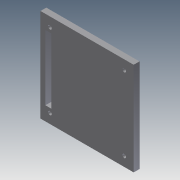
# Autodesk Inventor part: kinect rotate2 side
Saved by Autodesk Inventor 2011 (Build 150239000, 239)
## iProperties
Created: 2011-09-17
Part Number: kinect rotate2 side
Document SubType Name: Modeling
Designer: Matthew
Density: 1 g/cm^3
Author: Matthew
Autodesk Inventor part; units mm, degrees
ref_plane "YZ Plane" through (0, 0, 0) normal (1, 0, 0) x (0, 1, 0)
ref_plane "XZ Plane" through (0, 0, 0) normal (0, 1, 0) x (-1, 0, 0)
ref_plane "XY Plane" through (0, 0, 0) normal (0, 0, 1) x (1, 0, 0)
sketch "Sketch1" plane through (0, 0, 0) normal (0, 0, 1) x (1, 0, 0)
  line L0 (-25.4072, 25.3665) -> (76.1928, 25.3665)
  line L1 (76.1928, 25.3665) -> (76.1928, -76.2335)
  line L2 (76.1928, -76.2335) -> (-25.4072, -76.2335)
  line L3 (-25.4072, -76.2335) -> (-25.4072, 25.3665)
  point P0 (0, 0)
  dimension "d0" = 101.6
  dimension "d1" = 101.6
  constraints: 8 end point, 2 parallel, 1 horizontal, 1 perpendicular
  measures "d0" distance of L1.end L2.end
  measures "d1" distance of L0.end L1.end
extrude "Extrusion1" add sketch "Sketch1" along normal blind 0.7366
sketch "Sketch2" plane through (0, 0, 0.7366) normal (0, 0, 1) x (1, 0, 0)
  line L0 (-25.4072, 25.3665) -> (76.1928, -76.2335)
  line L1 (76.1928, 25.3665) -> (-25.4072, -76.2335)
  circle A0 centre (25.3928, -25.4335) radius 27.432
  point P0 (0, 0)
  dimension "d4" = 54.864
  constraints: 4 end point, 1 centre point, 1 midpoint, 1 perpendicular
  measures "d4" diameter of A0
extrude "Extrusion2" cut sketch "Sketch2" against normal blind 0.7366
sketch "Sketch3" plane through (0, 0, 0.7366) normal (0, 0, 1) x (1, 0, 0)
  line L0 (-25.4072, -76.2335) -> (-25.4072, 25.3665) projected
  line L1 (-25.4072, 25.3665) -> (-25.4072, -25.4335)
  line L2 (-25.4072, -25.4335) -> (-25.4072, 19.4102)
  line L3 (-25.4072, 25.3665) -> (76.1928, -76.2335)
  line L4 (76.1928, 25.3665) -> (-25.4072, -76.2335)
  circle A0 centre (-19.4509, 19.4102) radius 1.9812
  point P0 (0, 0)
  dimension "d7" = 44.8437
  dimension "d8" = 3.9624
  constraints: 8 end point, 2 point on line, 1 centre point, 1 midpoint, 1 perpendicular
  measures "d7" distance of L1.end L2.end
  measures "d8" diameter of A0
extrude "Extrusion3" cut sketch "Sketch3" against normal blind 0.7366 contours A0 L3 | L3 A0
sketch "Sketch4" plane through (0, 0, 0.7366) normal (0, 0, 1) x (1, 0, 0)
  line L0 (-25.4072, -76.2335) -> (76.1928, 25.3665)
  line L1 (-25.4072, 25.3665) -> (76.1928, -76.2335)
  circle A0 centre (70.2365, 19.4102) radius 1.9819
  circle A1 centre (70.2365, -70.2772) radius 1.983
  circle A2 centre (-19.4509, -70.2772) radius 1.9812
  point P0 (0, 0)
  constraints: 4 end point, 3 centre point, 3 point on line, 1 perpendicular
extrude "Extrusion4" cut sketch "Sketch4" against normal blind 0.7366
sketch "Sketch5" plane through (0, 0, 0.7366) normal (0, 0, 1) x (1, 0, 0)
  circle A0 centre (25.3928, -25.4335) radius 27.432 projected
  circle A1 centre (25.3928, -25.4335) radius 29.972
  circle A2 centre (25.3928, -25.4335) radius 32.512
  point P0 (0, 0)
  dimension "d13" = 59.944
  dimension "d14" = 65.024
  constraints: 2 centre point, 2 coincident
  measures "d13" diameter of A1
  measures "d14" diameter of A2
extrude "Extrusion5" add sketch "Sketch5" along normal blind 6.6548 contours A2
fillet "Fillet1" radius 3.175 4 edges at (-25.4072, 25.3665, 0.3683) (76.1928, 25.3665, 0.3683) (76.1928, -76.2335, 0.3683) (-25.4072, -76.2335, 0.3683)
sketch "Sketch6" plane through (25.3928, -25.4335, 0.7366) normal (0, 0, 1) x (1, 0, 0)
  circle A0 centre (0, 0) radius 29.972 projected
  circle A1 centre (0, 0) radius 27.432 projected
  point P0 (-25.3928, 25.4335)
extrude "Extrusion6" add sketch "Sketch6" along normal blind 9.1948
sketch "Sketch7" plane through (25.3928, -25.4335, 7.3914) normal (0, 0, 1) x (1, 0, 0)
  circle A0 centre (0, 0) radius 29.972 projected
  circle A1 centre (0, 0) radius 32.512 projected
  point P0 (-25.3928, 25.4335)
extrude "Extrusion7" cut sketch "Sketch7" against normal blind 6.6548
sketch "Sketch8" plane through (25.3928, -25.4335, 9.9314) normal (0, 0, 1) x (1, 0, 0)
  circle A0 centre (0, 0) radius 27.432 projected
  circle A1 centre (0, 0) radius 29.972 projected
  point P0 (-25.3928, 25.4335)
extrude "Extrusion8" cut sketch "Sketch8" against normal blind 2.54
sketch "Sketch9" plane through (0, 0, 0.7366) normal (0, 0, 1) x (1, 0, 0)
  circle A0 centre (-19.4509, 19.4102) radius 1.9812 projected
  circle A1 centre (70.2365, -70.2772) radius 1.983 projected
  circle A2 centre (-19.4509, -70.2772) radius 1.9812 projected
  circle A3 centre (70.2365, 19.4102) radius 1.9819 projected
  point P0 (0, 0)
extrude "Extrusion9" add sketch "Sketch9" against normal blind 0.7366
sketch "Sketch10" plane through (0, 0, 0.7366) normal (0, 0, 1) x (1, 0, 0)
  line L0 (-25.4072, 25.3665) -> (76.1928, 25.3665)
  line L1 (76.1928, 25.3665) -> (76.1928, -76.2335)
  line L2 (76.1928, -76.2335) -> (-25.4072, -76.2335)
  line L3 (-25.4072, -76.2335) -> (-25.4072, 25.3665)
  line L4 (-25.4072, 25.3665) -> (76.1928, -76.2335)
  line L5 (-25.4072, -76.2335) -> (76.1928, 25.3665)
  line L6 (-25.4072, 25.3665) -> (-25.4072, -25.4335)
  line L7 (-25.4072, -25.4335) -> (-25.4072, 15.0541)
  circle A0 centre (-15.0948, 15.0541) radius 1.9812
  circle A1 centre (65.8804, 15.0541) radius 1.9818
  circle A2 centre (65.8804, -65.9211) radius 1.9832
  circle A3 centre (-15.0948, -65.9211) radius 1.9812
  point P0 (0, 0)
  dimension "d26" = 40.4876
  dimension "d27" = 3.9624
  constraints: 16 end point, 5 point on line, 4 centre point, 2 parallel, 2 perpendicular, 1 horizontal, 1 midpoint
  measures "d26" distance of L6.end L7.end
  measures "d27" diameter of A0
extrude "Extrusion10" cut sketch "Sketch10" against normal blind 0.7366 contours A0 L4 | L4 A0 | A1 L5 | L5 A1 | A2 L4 | L4 A2 | A3 L5 | L5 A3
sketch "Sketch11" plane through (0, 0, 0.7366) normal (0, 0, 1) x (1, 0, 0)
  circle A0 centre (-15.0948, 15.0541) radius 1.9812 projected
  circle A1 centre (-15.0948, -65.9211) radius 1.9812 projected
  circle A2 centre (65.8804, 15.0541) radius 1.9818 projected
  circle A3 centre (65.8804, -65.9211) radius 1.9832 projected
  line L0 (-25.4072, 25.3665) -> (76.1928, 25.3665)
  line L1 (76.1928, 25.3665) -> (76.1928, -76.2335)
  line L2 (76.1928, -76.2335) -> (-25.4072, -76.2335)
  line L3 (-25.4072, -76.2335) -> (-25.4072, 25.3665)
  point P0 (0, 0)
  constraints: 8 end point, 2 parallel, 1 horizontal, 1 perpendicular
extrude "Extrusion11" add sketch "Sketch11" along normal blind 12.7
sketch "Sketch12" plane through (0, 0, 13.4366) normal (0, 0, 1) x (1, 0, 0)
  circle A0 centre (65.8804, -65.9211) radius 1.9832 projected
  circle A1 centre (65.8804, 15.0541) radius 1.9818 projected
  circle A2 centre (-15.0948, 15.0541) radius 1.9812 projected
  circle A3 centre (-15.0948, -65.9211) radius 1.9812 projected
  line L0 (76.1928, 25.3665) -> (76.1928, -76.2335) projected
  line L1 (-25.4072, 25.3665) -> (76.1928, 25.3665) projected
  line L2 (-25.4072, -76.2335) -> (-25.4072, 25.3665) projected
  line L3 (76.1928, -76.2335) -> (-25.4072, -76.2335) projected
  point P0 (0, 0)
extrude "Extrusion12" add sketch "Sketch12" against normal blind 19.05
sketch "Sketch13" plane through (0, 0, 13.4366) normal (0, 0, 1) x (1, 0, 0)
  circle A0 centre (65.8804, -65.9211) radius 1.9832 projected
  circle A1 centre (65.8804, 15.0541) radius 1.9818 projected
  circle A2 centre (-15.0948, 15.0541) radius 1.9812 projected
  circle A3 centre (-15.0948, -65.9211) radius 1.9812 projected
  line L0 (76.1928, 25.3665) -> (76.1928, -76.2335) projected
  line L1 (-25.4072, 25.3665) -> (76.1928, 25.3665) projected
  line L2 (-25.4072, -76.2335) -> (-25.4072, 25.3665) projected
  line L3 (76.1928, -76.2335) -> (-25.4072, -76.2335) projected
  point P0 (0, 0)
extrude "Extrusion13" cut sketch "Sketch13" against normal blind 12.7
sketch "Sketch14" plane through (-25.4072, 25.3665, -5.6134) normal (0, 1, 0) x (1, 0, 0)
  line L0 (0, -6.35) -> (101.6, -6.35) projected
  line L1 (101.6, -6.35) -> (101.6, 0) projected
  line L2 (101.6, 0) -> (0, 0) projected
  line L3 (0, 0) -> (0, -6.35) projected
  point P0 (25.4072, -5.6134)
sketch "Sketch15" plane through (-25.4072, -76.2335, -5.6134) normal (-1, 0, 0) x (0, 0, 1)
  line L0 (6.35, 0) -> (6.35, 101.6) projected
  line L1 (0, 101.6) -> (6.35, 101.6) projected
  line L2 (0, 101.6) -> (0, 0) projected
  line L3 (6.35, 0) -> (0, 0) projected
  point P0 (5.6134, 76.2335)
sketch "Sketch16" plane through (-25.4072, -76.2335, -5.6134) normal (0, -1, 0) x (1, 0, 0)
  line L0 (101.6, 6.35) -> (0, 6.35) projected
  line L1 (0, 6.35) -> (0, 0) projected
  line L2 (0, 0) -> (101.6, 0) projected
  line L3 (101.6, 6.35) -> (101.6, 0) projected
  point P0 (25.4072, 5.6134)
sketch "Sketch17" plane through (76.1928, -76.2335, -5.6134) normal (1, 0, 0) x (0, 0, -1)
  line L0 (-6.35, 101.6) -> (-6.35, 0) projected
  line L1 (-6.35, 0) -> (0, 0) projected
  line L2 (0, 0) -> (0, 101.6) projected
  line L3 (-6.35, 101.6) -> (0, 101.6) projected
  point P0 (-5.6134, 76.2335)
extrude "Extrusion14" add sketch "Sketch14" along normal blind 53.975
extrude "Extrusion15" add sketch "Sketch17" along normal blind 47.625
extrude "Extrusion16" add sketch "Sketch16" along normal blind 47.625
extrude "Extrusion17" add sketch "Sketch15" along normal blind 53.975
sketch "Sketch18" plane through (-25.4072, 25.3665, 0.7366) normal (0, 1, 0) x (1, 0, 0)
  line L0 (-53.975, 6.35) -> (-53.975, 0) projected
  line L1 (0, 0) -> (-53.975, 0) projected
  line L2 (0, 6.35) -> (0, 0) projected
  line L3 (0, 6.35) -> (-53.975, 6.35) projected
  point P0 (25.4072, 0.7366)
extrude "Extrusion18" add sketch "Sketch18" along normal blind 53.975
sketch "Sketch19" plane through (76.1928, 25.3665, 0.7366) normal (0, 1, 0) x (1, 0, 0)
  line L0 (47.625, 0) -> (47.625, 6.35) projected
  line L1 (0, 6.35) -> (47.625, 6.35) projected
  line L2 (0, 0) -> (0, 6.35) projected
  line L3 (0, 0) -> (47.625, 0) projected
  point P0 (-76.1928, 0.7366)
extrude "Extrusion19" add sketch "Sketch19" along normal blind 53.975
sketch "Sketch20" plane through (-25.4072, -123.8585, -5.6134) normal (-1, 0, 0) x (0, 0, 1)
  line L0 (6.35, 47.625) -> (0, 47.625) projected
  line L1 (0, 47.625) -> (0, 0) projected
  line L2 (0, 0) -> (6.35, 0) projected
  line L3 (6.35, 0) -> (6.35, 47.625) projected
  point P0 (5.6134, 123.8585)
extrude "Extrusion20" add sketch "Sketch20" along normal blind 53.975
sketch "Sketch21" plane through (123.8178, -76.2335, -5.6134) normal (0, -1, 0) x (1, 0, 0)
  line L0 (-47.625, 6.35) -> (-47.625, 0) projected
  line L1 (-47.625, 0) -> (0, 0) projected
  line L2 (0, 0) -> (0, 6.35) projected
  line L3 (0, 6.35) -> (-47.625, 6.35) projected
  point P0 (-123.8178, 5.6134)
extrude "Extrusion21" add sketch "Sketch21" along normal blind 47.625
sketch "Sketch22" plane through (-25.4072, 79.3415, -5.6134) normal (0, 1, 0) x (1, 0, 0)
  line L0 (149.225, -6.35) -> (-53.975, -6.35) projected
  line L1 (149.225, 0) -> (149.225, -6.35) projected
  line L2 (-53.975, 0) -> (149.225, 0) projected
  line L3 (-53.975, -6.35) -> (-53.975, 0) projected
  point P0 (25.4072, -5.6134)
extrude "Extrusion22" cut sketch "Sketch22" against normal blind 53.975
sketch "Sketch23" plane through (-79.3822, -76.2335, -5.6134) normal (-1, 0, 0) x (0, 0, 1)
  line L0 (6.35, 101.6) -> (0, 101.6) projected
  line L1 (0, -47.625) -> (0, 101.6) projected
  line L2 (6.35, -47.625) -> (0, -47.625) projected
  line L3 (6.35, 101.6) -> (6.35, -47.625) projected
  point P0 (5.6134, 76.2335)
extrude "Extrusion23" cut sketch "Sketch23" against normal blind 53.975
sketch "Sketch24" plane through (-25.4072, -123.8585, -5.6134) normal (0, -1, 0) x (1, 0, 0)
  line L0 (0, 6.35) -> (0, 0) projected
  line L1 (149.225, 0) -> (0, 0) projected
  line L2 (149.225, 6.35) -> (149.225, 0) projected
  line L3 (0, 6.35) -> (149.225, 6.35) projected
  point P0 (25.4072, 5.6134)
extrude "Extrusion24" cut sketch "Sketch24" against normal blind 47.625
sketch "Sketch25" plane through (123.8178, -76.2335, -5.6134) normal (1, 0, 0) x (0, 0, -1)
  line L0 (-6.35, 0) -> (0, 0) projected
  line L1 (0, 101.6) -> (0, 0) projected
  line L2 (0, 101.6) -> (-6.35, 101.6) projected
  line L3 (-6.35, 0) -> (-6.35, 101.6) projected
  point P0 (-5.6134, 76.2335)
extrude "Extrusion25" cut sketch "Sketch25" against normal blind 47.625
sketch "Sketch26" plane through (-25.4072, 25.3665, -5.6134) normal (0, 1, 0) x (1, 0, 0)
  line L0 (101.6, -6.35) -> (101.6, 0) projected
  line L1 (0, 0) -> (101.6, 0) projected
  line L2 (0, 0) -> (0, -6.35) projected
  line L3 (101.6, -6.35) -> (0, -6.35) projected
  point P0 (25.4072, -5.6134)
extrude "Extrusion26" add sketch "Sketch26" along normal blind 53.975
sketch "Sketch27" plane through (-25.4072, -76.2335, -5.6134) normal (-1, 0, 0) x (0, 0, 1)
  line L0 (0, 0) -> (6.35, 0) projected
  line L1 (6.35, 0) -> (6.35, 155.575) projected
  line L2 (6.35, 155.575) -> (0, 155.575) projected
  line L3 (0, 0) -> (0, 155.575) projected
  point P0 (5.6134, 76.2335)
extrude "Extrusion27" add sketch "Sketch27" along normal blind 53.975
sketch "Sketch28" plane through (-25.4072, -76.2335, -5.6134) normal (0, -1, 0) x (1, 0, 0)
  line L0 (101.6, 0) -> (101.6, 6.35) projected
  line L1 (101.6, 6.35) -> (-53.975, 6.35) projected
  line L2 (-53.975, 6.35) -> (-53.975, 0) projected
  line L3 (101.6, 0) -> (-53.975, 0) projected
  point P0 (25.4072, 5.6134)
extrude "Extrusion28" add sketch "Sketch28" along normal blind 22.225
sketch "Sketch29" plane through (-25.4072, 79.3415, -5.6134) normal (0, 1, 0) x (1, 0, 0)
  line L0 (101.6, -6.35) -> (-53.975, -6.35) projected
  line L1 (101.6, 0) -> (101.6, -6.35) projected
  line L2 (-53.975, 0) -> (101.6, 0) projected
  line L3 (-53.975, 0) -> (-53.975, -6.35) projected
  point P0 (25.4072, -5.6134)
extrude "Extrusion29" add sketch "Sketch29" along normal blind 158.6992
sketch "Sketch30" plane through (-25.4072, 238.0407, -5.6134) normal (0, 1, 0) x (1, 0, 0)
  line L0 (-53.975, -6.35) -> (-53.975, 0) projected
  line L1 (101.6, -6.35) -> (-53.975, -6.35) projected
  line L2 (101.6, 0) -> (101.6, -6.35) projected
  line L3 (-53.975, 0) -> (101.6, 0) projected
  point P0 (25.4072, -5.6134)
extrude "Extrusion30" add sketch "Sketch30" along normal blind 177.8
sketch "Sketch31" plane through (0, 0, 0.7366) normal (0, 0, 1) x (1, 0, 0)
  line L0 (76.1928, 415.8407) -> (76.1928, -98.4585) projected
  line L1 (76.1928, 415.8407) -> (-79.3822, 415.8407) projected
  line L2 (65.8804, 415.8407) -> (65.8804, 383.3033)
  line L3 (65.8804, 383.3033) -> (-17.076, 383.3033)
  line L4 (-17.076, 383.3033) -> (-13.1136, 383.3033)
  line L5 (-13.1136, 383.3033) -> (-15.0948, 383.3033)
  circle A0 centre (-15.0948, 383.3033) radius 1.9812
  circle A1 centre (65.8804, 383.3033) radius 1.9812
  line L6 (65.8804, 383.3033) -> (65.8804, 302.3281)
  circle A2 centre (65.8804, 302.3281) radius 1.9812
  line L7 (-15.0948, 383.3033) -> (-15.0948, 302.3281)
  circle A3 centre (-15.0948, 302.3281) radius 1.9812
  point P0 (0, 0)
  dimension "d70" = 32.5374
  dimension "d71" = 80.9752
  constraints: 12 end point, 4 coincident, 3 centre point, 2 parallel, 2 perpendicular, 2 point on line, 1 horizontal alignment, 1 midpoint, 2 other
  measures "d70" distance of L2.start L2.end
  measures "d71" distance of L6.start L6.end
extrude "Extrusion31" cut sketch "Sketch31" against normal blind 177.8
sketch "Sketch32" plane through (0, 0, -5.6134) normal (0, 0, -1) x (-1, 0, 0)
  circle A0 centre (15.0948, 383.3033) radius 1.9812 projected
  circle A1 centre (15.0948, 302.3281) radius 1.9812 projected
  circle A2 centre (-65.8804, 302.3281) radius 1.9812 projected
  circle A3 centre (-65.8804, 383.3033) radius 1.9812 projected
  circle A4 centre (15.0948, -65.9211) radius 1.9812 projected
  circle A5 centre (15.0948, 15.0541) radius 1.9812 projected
  circle A6 centre (-65.8804, 15.0541) radius 1.9818 projected
  circle A7 centre (-65.8804, -65.9211) radius 1.9832 projected
  line L0 (-76.1928, 415.8407) -> (-76.1928, -98.4585) projected
  line L1 (-76.1928, -98.4585) -> (79.3822, -98.4585) projected
  line L2 (79.3822, -98.4585) -> (79.3822, 415.8407) projected
  line L3 (79.3822, 415.8407) -> (-76.1928, 415.8407) projected
  point P0 (0, 0)
extrude "Extrusion32" add sketch "Sketch32" along normal blind 6.35
sketch "Sketch33" plane through (0, 0, 0.7366) normal (0, 0, 1) x (1, 0, 0)
  line L0 (76.1928, 415.8407) -> (76.1928, -98.4585) projected
  line L1 (76.1928, 158.6911) -> (76.1928, 107.8911)
  line L2 (76.1928, 107.8911) -> (25.3928, 107.8911)
  line L3 (25.3928, 107.8911) -> (25.3928, 209.4911)
  line L4 (25.3928, 209.4911) -> (76.1928, 209.4911)
  line L5 (76.1928, 209.4911) -> (76.1928, 107.8911)
  point P0 (0, 0)
  dimension "d76" = 50.8
  dimension "d77" = 50.8
  dimension "d78" = 101.6
  constraints: 10 end point, 2 parallel, 1 horizontal, 1 midpoint, 1 perpendicular, 1 point on line
  measures "d76" distance of L1.start L1.end
  measures "d77" distance of L3.end L4.end
  measures "d78" distance of L2.end L3.end
extrude "Extrusion33" cut sketch "Sketch33" against normal blind 25.4
sketch "Sketch34" plane through (0, 0, 0.7366) normal (0, 0, 1) x (1, 0, 0)
  line L0 (25.3928, 107.8911) -> (25.3928, 209.4911) projected
  line L1 (76.1928, 107.8911) -> (76.1928, -98.4585) projected
  line L2 (25.3928, 158.6911) -> (-25.4072, 158.6911)
  circle A0 centre (-25.4072, 158.6911) radius 12.7
  point P0 (0, 0)
  dimension "d81" = 50.8
  dimension "d82" = 25.4
  constraints: 2 end point, 1 centre point, 1 coincident, 1 midpoint, 1 perpendicular
  measures "d81" distance of L2.start L2.end
  measures "d82" diameter of A0
extrude "Extrusion34" cut sketch "Sketch34" against normal blind 25.4
fillet "Fillet2" radius 12.7 2 edges at (25.3928, 209.4911, -5.6134) (25.3928, 107.8911, -5.6134)
sketch "Sketch35" plane through (0, 0, 0.7366) normal (0, 0, 1) x (1, 0, 0)
  line L0 (-79.3822, 415.8407) -> (76.1928, 415.8407)
  line L1 (76.1928, 415.8407) -> (76.1928, 422.1907)
  line L2 (76.1928, 422.1907) -> (-79.3822, 422.1907)
  line L3 (-79.3822, 422.1907) -> (-79.3822, 415.8407)
  line L4 (-79.3822, -98.4585) -> (76.1928, -98.4585)
  line L5 (76.1928, -98.4585) -> (76.1928, -104.8085)
  line L6 (76.1928, -104.8085) -> (-79.3822, -104.8085)
  line L7 (-79.3822, -104.8085) -> (-79.3822, -98.4585)
  point P0 (0, 0)
  dimension "d86" = 6.35
  dimension "d87" = 6.35
  constraints: 16 end point, 4 parallel, 2 horizontal, 2 perpendicular
  measures "d86" distance of L1.end L0.end
  measures "d87" distance of L4.end L5.end
extrude "Extrusion35" add sketch "Sketch35" against normal blind 6.35
sketch "Sketch36" plane through (-25.4072, 415.8407, -5.6134) normal (0, 1, 0) x (1, 0, 0)
  line L0 (-53.975, 0) -> (101.6, 0) projected
  line L1 (101.6, 6.35) -> (101.6, 0) projected
  line L2 (101.6, 6.35) -> (-53.975, 6.35) projected
  line L3 (-53.975, 0) -> (-53.975, 6.35) projected
  point P0 (25.4072, -5.6134)
extrude "Extrusion36" add sketch "Sketch36" along normal blind 6.35
sketch "Sketch37" plane through (-25.4072, -98.4585, -5.6134) normal (0, -1, 0) x (1, 0, 0)
  line L0 (101.6, 0) -> (-53.975, 0) projected
  line L1 (-53.975, -6.35) -> (-53.975, 0) projected
  line L2 (-53.975, -6.35) -> (101.6, -6.35) projected
  line L3 (101.6, 0) -> (101.6, -6.35) projected
  point P0 (25.4072, 5.6134)
extrude "Extrusion37" add sketch "Sketch37" along normal blind 6.35
sketch "Sketch38" plane through (0, 0, 0.7366) normal (0, 0, 1) x (1, 0, 0)
  line L0 (76.1928, 422.1907) -> (-79.3822, 422.1907) projected
  line L1 (76.1928, 107.8911) -> (76.1928, -104.8085) projected
  circle A0 centre (65.8804, 302.3281) radius 1.9812 projected
  circle A1 centre (-15.0948, 302.3281) radius 1.9812 projected
  line L2 (-15.0948, 422.1907) -> (-15.0948, 405.5283)
  line L3 (-15.0948, 405.5283) -> (65.8804, 405.5283)
  line L4 (65.8804, 302.3281) -> (65.8804, 324.5531)
  line L5 (-15.0948, 302.3281) -> (-15.0948, 324.5531)
  circle A2 centre (-15.0948, 324.5531) radius 1.9812
  circle A3 centre (-15.0948, 405.5283) radius 1.9812
  circle A4 centre (65.8804, 405.5283) radius 1.9812
  circle A5 centre (65.8804, 324.5531) radius 1.9812
  point P0 (0, 0)
  dimension "d94" = 16.6624
  dimension "d95" = 22.225
  constraints: 8 end point, 4 centre point, 4 coincident, 3 parallel, 1 perpendicular, 1 point on line
  measures "d94" distance of L2.start L2.end
  measures "d95" distance of L4.start L4.end
extrude "Extrusion38" cut sketch "Sketch38" against normal blind 12.7 contours A3 L3 L2 | L2 L3 A3 | A2 | A4 | A5
sketch "Sketch39" plane through (0, 0, 0.7366) normal (0, 0, 1) x (1, 0, 0)
  circle A0 centre (65.8804, 383.3033) radius 1.9812 projected
  circle A1 centre (65.8804, 302.3281) radius 1.9812 projected
  circle A2 centre (-15.0948, 302.3281) radius 1.9812 projected
  circle A3 centre (-15.0948, 383.3033) radius 1.9812 projected
  point P0 (0, 0)
extrude "Extrusion39" add sketch "Sketch39" against normal blind 12.7
sketch "Sketch40" plane through (0, 0, 0.7366) normal (0, 0, 1) x (1, 0, 0)
  circle A0 centre (-15.0948, 15.0541) radius 1.9812 projected
  circle A1 centre (-15.0948, -65.9211) radius 1.9812 projected
  line L0 (76.1928, 107.8911) -> (76.1928, -104.8085) projected
  line L1 (-15.0948, -65.9211) -> (-15.0948, -88.1461)
  line L2 (-15.0948, -88.1461) -> (65.8804, -88.1461)
  line L3 (-15.0948, 15.0541) -> (-15.0948, -7.1709)
  line L4 (-15.0948, -7.1709) -> (65.8804, -7.1709)
  circle A2 centre (-15.0948, -88.1461) radius 1.9812
  circle A3 centre (65.8804, -88.1461) radius 1.9818
  circle A4 centre (65.8804, -7.1709) radius 1.9818
  circle A5 centre (-15.0948, -7.1709) radius 1.9812
  point P0 (0, 0)
  dimension "d100" = 22.225
  dimension "d101" = 22.225
  constraints: 8 end point, 4 centre point, 4 coincident, 3 perpendicular, 1 parallel
  measures "d100" distance of L1.start L1.end
  measures "d101" distance of L3.start L3.end
extrude "Extrusion40" cut sketch "Sketch40" against normal blind 12.7 contours A2 L2 L1 | L1 L2 A2 | A5 L4 L3 | L3 L4 A5 | A3 | A4
sketch "Sketch41" plane through (0, 0, 0.7366) normal (0, 0, 1) x (1, 0, 0)
  circle A0 centre (65.8804, -65.9211) radius 1.9832 projected
  circle A1 centre (65.8804, 15.0541) radius 1.9818 projected
  circle A2 centre (-15.0948, 15.0541) radius 1.9812 projected
  circle A3 centre (-15.0948, -65.9211) radius 1.9812 projected
  point P0 (0, 0)
extrude "Extrusion41" add sketch "Sketch41" against normal blind 12.7
sketch "Sketch42" plane through (0, 0, 0.7366) normal (0, 0, 1) x (1, 0, 0)
  circle A0 centre (65.8804, -7.1709) radius 1.9818 projected
  circle A1 centre (65.8804, -88.1461) radius 1.9818 projected
  circle A2 centre (-15.0948, -7.1709) radius 1.9812 projected
  circle A3 centre (-15.0948, -88.1461) radius 1.9812 projected
  circle A4 centre (-15.0948, 405.5283) radius 1.9812 projected
  circle A5 centre (-15.0948, 324.5531) radius 1.9812 projected
  circle A6 centre (65.8804, 405.5283) radius 1.9812 projected
  circle A7 centre (-25.4072, 158.6911) radius 12.7 projected
  line L0 (76.1928, 107.8911) -> (38.0928, 107.8911) projected
  arc A8 (25.3928, 120.5911) -> (38.0928, 107.8911) centre (38.0928, 120.5911) ccw projected
  line L1 (25.3928, 120.5911) -> (25.3928, 196.7911) projected
  arc A9 (38.0928, 209.4911) -> (25.3928, 196.7911) centre (38.0928, 196.7911) ccw projected
  line L2 (38.0928, 209.4911) -> (76.1928, 209.4911) projected
  line L3 (76.1928, 422.1907) -> (76.1928, 209.4911) projected
  line L4 (76.1928, 422.1907) -> (-79.3822, 422.1907) projected
  line L5 (-79.3822, 422.1907) -> (-79.3822, -104.8085) projected
  line L6 (-79.3822, -104.8085) -> (76.1928, -104.8085) projected
  line L7 (76.1928, 107.8911) -> (76.1928, -104.8085) projected
  line L8 (65.8804, 405.5283) -> (-15.0948, 405.5283)
  line L9 (-15.0948, 405.5283) -> (-15.0948, 324.5531)
  line L10 (25.3928, 365.0407) -> (25.3928, 415.8407)
  line L11 (25.3928, 415.8407) -> (-25.4072, 415.8407)
  line L12 (-25.4072, 415.8407) -> (76.1928, 415.8407)
  line L13 (76.1928, 415.8407) -> (76.1928, 314.2407)
  line L14 (76.1928, 314.2407) -> (-25.4072, 314.2407)
  line L15 (-25.4072, 314.2407) -> (-25.4072, 415.8407)
  point P0 (0, 0)
  dimension "d106" = 50.8
  dimension "d107" = 50.8
  dimension "d108" = 101.6
  dimension "d109" = 101.6
  constraints: 16 end point, 4 perpendicular, 3 parallel, 1 horizontal
  measures "d106" distance of L10.start L10.end
  measures "d107" distance of L10.end L11.end
  measures "d108" distance of L13.end L14.end
  measures "d109" distance of L12.end L13.end
extrude "Extrusion42" cut sketch "Sketch42" against normal blind 25.4 contours L7 L6 L5 L4 L3 L12 L11 L15 L14 L2 A9 L1 A8 L0
sketch "Sketch43" plane through (0, 0, 0.7366) normal (0, 0, 1) x (1, 0, 0)
  line L0 (-25.4072, 314.2407) -> (76.1928, 314.2407) projected
  line L1 (76.1928, 415.8407) -> (76.1928, 314.2407) projected
  line L2 (76.1928, 415.8407) -> (-25.4072, 415.8407) projected
  line L3 (-25.4072, 415.8407) -> (-25.4072, 314.2407) projected
  circle A0 centre (-15.0948, 405.5283) radius 1.9812 projected
  circle A1 centre (-15.0948, 324.5531) radius 1.9812 projected
  circle A2 centre (65.8804, 324.5531) radius 1.9812 projected
  circle A3 centre (65.8804, 405.5283) radius 1.9812 projected
  point P0 (0, 0)
extrude "Extrusion43" cut sketch "Sketch43" against normal blind 6.35
sketch "Sketch44" plane through (-25.4072, 415.8407, -11.9634) normal (0, 1, 0) x (1, 0, 0)
  line L0 (0, -6.35) -> (101.6, -6.35) projected
  line L1 (101.6, 0) -> (101.6, -6.35) projected
  line L2 (0, 0) -> (101.6, 0) projected
  line L3 (0, -6.35) -> (0, 0) projected
  point P0 (25.4072, -11.9634)
extrude "Extrusion44" add sketch "Sketch44" along normal blind 19.05
sketch "Sketch45" plane through (-25.4072, 314.2407, -11.9634) normal (0, -1, 0) x (1, 0, 0)
  line L0 (101.6, 6.35) -> (0, 6.35) projected
  line L1 (0, 6.35) -> (0, 0) projected
  line L2 (101.6, 0) -> (0, 0) projected
  line L3 (101.6, 6.35) -> (101.6, 0) projected
  point P0 (25.4072, 11.9634)
extrude "Extrusion45" add sketch "Sketch45" along normal blind 19.05
sketch "Sketch46" plane through (0, 0, -11.9634) normal (0, 0, -1) x (-1, 0, 0)
  line L0 (-76.1928, 295.1907) -> (25.4072, 295.1907) projected
  circle A0 centre (-65.8804, 324.5531) radius 1.9812 projected
  circle A1 centre (15.0948, 324.5531) radius 1.9812 projected
  circle A2 centre (15.0948, 405.5283) radius 1.9812 projected
  line L1 (-65.8804, 324.5531) -> (15.0948, 324.5531)
  line L2 (15.0948, 324.5531) -> (15.0948, 405.5283)
  circle A3 centre (-25.3928, 365.0407) radius 11.5
  line L3 (-25.3928, 365.0407) -> (-35.8928, 365.0407)
  line L4 (-35.8928, 365.0407) -> (-14.8928, 365.0407)
  line L5 (-14.8928, 365.0407) -> (-14.8928, 400.0407)
  line L6 (-14.8928, 400.0407) -> (-35.8928, 400.0407)
  line L7 (-35.8928, 400.0407) -> (-35.8928, 365.0407)
  point P0 (0, 0)
  dimension "d118" = 23
  dimension "d119" = 10.5
  dimension "d120" = 21
  dimension "d121" = 35
  constraints: 14 end point, 3 parallel, 3 perpendicular, 1 centre point, 1 horizontal
  measures "d118" diameter of A3
  measures "d119" distance of L3.start L3.end
  measures "d120" distance of L6.end L5.end
  measures "d121" distance of L5.end L4.end
extrude "Extrusion46" cut sketch "Sketch46" against normal blind 19.05 contours A3 L7 L3 L4 L5 | L5 L4 L3 L7 A3 | A3 L7 L6 L5
sketch "Sketch47" plane through (0, 0, -11.9634) normal (0, 0, -1) x (-1, 0, 0)
  arc A0 (-35.8928, 369.7311) -> (-14.8928, 369.7311) centre (-25.3928, 365.0407) ccw projected
  line L0 (-76.1928, 295.1907) -> (25.4072, 295.1907) projected
  line L1 (-25.3928, 365.0407) -> (-38.8928, 365.0407)
  line L2 (-38.8928, 365.0407) -> (-38.8928, 371.5407)
  line L3 (-38.8928, 371.5407) -> (-38.8928, 379.5407)
  line L4 (-38.8928, 379.5407) -> (-38.8928, 387.5407)
  line L5 (-38.8928, 371.5407) -> (-11.8928, 371.5407)
  line L6 (-38.8928, 387.5407) -> (-11.8928, 387.5407)
  circle A1 centre (-38.8928, 371.5407) radius 1
  circle A2 centre (-38.8928, 387.5407) radius 1
  circle A3 centre (-11.8928, 371.5407) radius 1
  circle A4 centre (-11.8928, 387.5407) radius 1
  point P0 (0, 0)
  dimension "d124" = 13.5
  dimension "d125" = 6.5
  dimension "d126" = 8
  dimension "d127" = 8
  dimension "d128" = 27
  dimension "d129" = 27
  dimension "d130" = 2
  constraints: 12 end point, 4 centre point, 4 coincident, 2 collinear, 2 parallel, 2 perpendicular
  measures "d124" distance of L1.start L1.end
  measures "d125" distance of L1.end L2.end
  measures "d126" distance of L2.end L3.end
  measures "d127" distance of L3.end L4.end
  measures "d128" distance of L2.end L5.end
  measures "d129" distance of L4.end L6.end
  measures "d130" diameter of A1
extrude "Extrusion47" cut sketch "Sketch47" against normal blind 25.4
sketch "Sketch48" plane through (0, 0, -5.6134) normal (0, 0, 1) x (1, 0, 0)
  circle A0 centre (38.8928, 371.5407) radius 1 projected
  circle A1 centre (38.8928, 387.5407) radius 1 projected
  circle A2 centre (11.8928, 387.5407) radius 1 projected
  circle A3 centre (11.8928, 371.5407) radius 1 projected
  line L0 (35.8928, 400.0407) -> (35.8928, 369.7311) projected
  arc A4 (14.8928, 369.7311) -> (35.8928, 369.7311) centre (25.3928, 365.0407) ccw projected
  line L1 (14.8928, 369.7311) -> (14.8928, 400.0407) projected
  line L2 (14.8928, 400.0407) -> (35.8928, 400.0407) projected
  point P0 (0, 0)
extrude "Extrusion48" add sketch "Sketch48" against normal blind 6.35
sketch "Sketch49" plane through (0, 0, -5.6134) normal (0, 0, 1) x (1, 0, 0)
  circle A0 centre (65.8804, 324.5531) radius 1.9812 projected
  line L0 (76.1928, 434.8907) -> (76.1928, 295.1907) projected
  line L1 (-25.4072, 295.1907) -> (-25.4072, 434.8907) projected
  line L2 (-25.4072, 324.5531) -> (76.1928, 324.5531)
  line L3 (65.8804, 324.5531) -> (76.1928, 324.5531)
  line L4 (76.1928, 324.5531) -> (76.1928, 314.2407)
  line L5 (76.1928, 314.2407) -> (65.8804, 314.2407)
  line L6 (65.8804, 314.2407) -> (65.8804, 324.5531)
  line L7 (76.1928, 314.2407) -> (-25.4072, 314.2407)
  line L8 (-25.4072, 314.2407) -> (-25.4072, 415.8407)
  line L9 (-25.4072, 415.8407) -> (76.1928, 415.8407)
  line L10 (76.1928, 415.8407) -> (76.1928, 314.2407)
  line L11 (-25.4072, 415.8407) -> (76.1928, 415.8407)
  line L12 (76.1928, 415.8407) -> (76.1928, 434.8907)
  line L13 (76.1928, 434.8907) -> (-25.4072, 434.8907)
  line L14 (-25.4072, 434.8907) -> (-25.4072, 415.8407)
  line L15 (76.1928, 314.2407) -> (-25.4072, 314.2407)
  line L16 (-25.4072, 314.2407) -> (-25.4072, 295.1907)
  line L17 (-25.4072, 295.1907) -> (76.1928, 295.1907)
  line L18 (76.1928, 295.1907) -> (76.1928, 314.2407)
  point P0 (0, 0)
  dimension "d135" = 10.3124
  dimension "d136" = 101.6
  dimension "d137" = 101.6
  constraints: 34 end point, 8 parallel, 5 perpendicular, 4 horizontal, 3 point on line
  measures "d135" distance of L3.end L4.end
  measures "d136" distance of L8.end L9.end
  measures "d137" distance of L7.end L8.end
extrude "Extrusion49" cut sketch "Sketch49" against normal blind 6.35 contours L5 L0 L17 L1 L7 | L9 L1 L13 L0
sketch "Sketch50" plane through (0, 0, -11.9634) normal (0, 0, -1) x (-1, 0, 0)
  line L0 (-76.1928, 314.2407) -> (25.4072, 314.2407) projected
  line L1 (25.4072, 314.2407) -> (20.0732, 314.2407)
  line L2 (20.0732, 314.2407) -> (13.7232, 314.2407)
  line L3 (13.7232, 314.2407) -> (13.7232, 329.4807)
  line L4 (13.7232, 329.4807) -> (20.0732, 329.4807)
  line L5 (20.0732, 329.4807) -> (20.0732, 314.2407)
  line L6 (13.7232, 329.4807) -> (20.0732, 329.4807)
  line L7 (20.0732, 329.4807) -> (20.0732, 400.6007)
  line L8 (20.0732, 400.6007) -> (13.7232, 400.6007)
  line L9 (13.7232, 400.6007) -> (13.7232, 329.4807)
  point P0 (0, 0)
  dimension "d140" = 5.334
  dimension "d141" = 6.35
  dimension "d142" = 15.24
  dimension "d143" = 71.12
  constraints: 18 end point, 3 parallel, 3 perpendicular, 2 point on line, 1 horizontal
  measures "d140" distance of L0.end L1.end
  measures "d141" distance of L1.end L2.end
  measures "d142" distance of L2.end L3.end
  measures "d143" distance of L7.end L6.end
extrude "Extrusion50" cut sketch "Sketch50" against normal blind 6.35 contours L9 L8 L7 L4
sketch "Sketch51" plane through (0, 0, -11.9634) normal (0, 0, -1) x (-1, 0, 0)
  line L0 (13.7232, 329.4807) -> (20.0732, 329.4807)
  line L1 (20.0732, 329.4807) -> (20.0732, 328.7187)
  line L2 (20.0732, 328.7187) -> (13.7232, 328.7187)
  line L3 (13.7232, 328.7187) -> (13.7232, 329.4807)
  line L4 (13.7232, 400.6007) -> (20.0732, 400.6007)
  line L5 (20.0732, 400.6007) -> (20.0732, 401.3627)
  line L6 (20.0732, 401.3627) -> (13.7232, 401.3627)
  line L7 (13.7232, 401.3627) -> (13.7232, 400.6007)
  point P0 (0, 0)
  dimension "d146" = 0.762
  dimension "d147" = 0.762
  constraints: 16 end point, 4 parallel, 2 horizontal, 2 perpendicular
  measures "d146" distance of L0.end L1.end
  measures "d147" distance of L5.end L4.end
extrude "Extrusion51" cut sketch "Sketch51" against normal blind 6.35
sketch "Sketch52" plane through (0, 0, -5.6134) normal (0, 0, 1) x (1, 0, 0)
  circle A0 centre (65.8804, 324.5531) radius 1.9812 projected
  circle A1 centre (65.8804, 405.5283) radius 1.9812 projected
  circle A2 centre (-15.0948, 405.5283) radius 1.9812 projected
  circle A3 centre (-15.0948, 324.5531) radius 1.9812 projected
  line L0 (-15.0948, 405.5283) -> (65.8804, 324.5531)
  line L1 (-15.0948, 324.5531) -> (65.8804, 405.5283)
  circle A4 centre (25.3928, 365.0407) radius 8
  circle A5 centre (33.3928, 365.0407) radius 1
  circle A6 centre (25.3928, 357.0407) radius 1
  circle A7 centre (25.3928, 373.0407) radius 1
  circle A8 centre (17.3928, 365.0407) radius 1
  point P0 (0, 0)
  dimension "d150" = 16
  dimension "d151" = 2
  dimension "d152" = 2
  dimension "d153" = 2
  dimension "d154" = 2
  constraints: 5 centre point, 4 end point, 4 point on circle, 2 midpoint, 1 perpendicular
  measures "d150" diameter of A4
  measures "d151" diameter of A5
  measures "d152" diameter of A6
  measures "d153" diameter of A7
  measures "d154" diameter of A8
extrude "Extrusion52" cut sketch "Sketch52" against normal blind 6.35 contours A7 A4 | A4 A7 | A8 A4 | A4 A8 | A6 A4 | A4 A6 | A5 A4 | A4 A5
body "Solid1"
